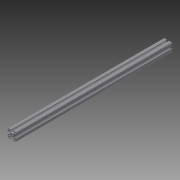
# Autodesk Inventor part: 28 piece
Saved by Autodesk Inventor 2013 (Build 170138000, 138)
## iProperties
Created: 2012-08-14
Part Number: 28 piece
Material: Generic
Document SubType Name: Modeling
Designer: Admin
Density: 1 g/cm^3
Author: Admin
Autodesk Inventor part; units mm, degrees
ref_plane "YZ Plane" through (0, 0, 0) normal (1, 0, 0) x (0, 1, 0)
ref_plane "XZ Plane" through (0, 0, 0) normal (0, 1, 0) x (-1, 0, 0)
ref_plane "XY Plane" through (0, 0, 0) normal (0, 0, 1) x (1, 0, 0)
sketch "Sketch1" plane through (0, 0, 0) normal (0, 0, 1) x (1, 0, 0)
  line L0 (19.5541, -5.1054) -> (14.9059, -5.1054)
  arc A0 (19.9351, -5.4864) -> (19.5541, -5.1054) centre (19.5541, -5.4864) ccw
  line L1 (19.9351, -7.7216) -> (19.9351, -5.4864)
  arc A1 (17.1411, -10.5156) -> (19.9351, -7.7216) centre (17.1411, -7.7216) ccw
  line L2 (14.9059, -10.5156) -> (17.1411, -10.5156)
  arc A2 (14.5249, -10.1346) -> (14.9059, -10.5156) centre (14.9059, -10.1346) ccw
  line L3 (14.5249, -5.4864) -> (14.5249, -10.1346)
  arc A3 (14.9059, -5.1054) -> (14.5249, -5.4864) centre (14.9059, -5.4864) ccw
  arc A4 (5.9905, 6.7564) -> (-0.6643, 6.7564) centre (2.6631, 6.7564) ccw
  arc A5 (-0.6643, 6.7564) -> (5.9905, 6.7564) centre (2.6631, 6.7564) ccw
  line L4 (17.1411, 24.0284) -> (14.9059, 24.0284)
  arc A6 (19.9351, 21.2344) -> (17.1411, 24.0284) centre (17.1411, 21.2344) ccw
  line L5 (19.9351, 18.9992) -> (19.9351, 21.2344)
  arc A7 (19.5541, 18.6182) -> (19.9351, 18.9992) centre (19.5541, 18.9992) ccw
  line L6 (14.9059, 18.6182) -> (19.5541, 18.6182)
  arc A8 (14.5249, 18.9992) -> (14.9059, 18.6182) centre (14.9059, 18.9992) ccw
  line L7 (14.5249, 23.6474) -> (14.5249, 18.9992)
  arc A9 (14.9059, 24.0284) -> (14.5249, 23.6474) centre (14.9059, 23.6474) ccw
  line L8 (-11.8149, -10.5156) -> (-9.5797, -10.5156)
  arc A10 (-14.6089, -7.7216) -> (-11.8149, -10.5156) centre (-11.8149, -7.7216) ccw
  line L9 (-14.6089, -5.4864) -> (-14.6089, -7.7216)
  arc A11 (-14.2279, -5.1054) -> (-14.6089, -5.4864) centre (-14.2279, -5.4864) ccw
  line L10 (-9.5797, -5.1054) -> (-14.2279, -5.1054)
  arc A12 (-9.1987, -5.4864) -> (-9.5797, -5.1054) centre (-9.5797, -5.4864) ccw
  line L11 (-9.1987, -10.1346) -> (-9.1987, -5.4864)
  arc A13 (-9.5797, -10.5156) -> (-9.1987, -10.1346) centre (-9.5797, -10.1346) ccw
  line L12 (-14.2279, 18.6182) -> (-9.5797, 18.6182)
  arc A14 (-14.6089, 18.9992) -> (-14.2279, 18.6182) centre (-14.2279, 18.9992) ccw
  line L13 (-14.6089, 21.2344) -> (-14.6089, 18.9992)
  arc A15 (-11.8149, 24.0284) -> (-14.6089, 21.2344) centre (-11.8149, 21.2344) ccw
  line L14 (-9.5797, 24.0284) -> (-11.8149, 24.0284)
  arc A16 (-9.1987, 23.6474) -> (-9.5797, 24.0284) centre (-9.5797, 23.6474) ccw
  line L15 (-9.1987, 18.9992) -> (-9.1987, 23.6474)
  arc A17 (-9.5797, 18.6182) -> (-9.1987, 18.9992) centre (-9.5797, 18.9992) ccw
  arc A18 (-7.6239, 19.5366) -> (-7.3636, 18.9083) centre (-6.7353, 19.5366) ccw
  line L16 (-7.6239, 19.5366) -> (-7.6239, 21.3111)
  arc A19 (-6.3539, 22.5811) -> (-7.6239, 21.3111) centre (-6.3539, 21.3111) ccw
  line L17 (-6.3539, 22.5811) -> (-4.151, 22.5811)
  line L18 (-4.151, 22.5811) -> (-4.151, 21.7424)
  line L19 (-4.151, 21.7424) -> (-2.9757, 21.7424)
  arc A20 (-2.9757, 21.7424) -> (-1.4009, 23.3172) centre (-2.9757, 23.3172) ccw
  line L20 (-1.4009, 23.3172) -> (-1.4009, 24.2316)
  arc A21 (-1.4009, 24.2316) -> (-2.9757, 25.8064) centre (-2.9757, 24.2316) ccw
  line L21 (-2.9757, 25.8064) -> (-5.3125, 25.8064)
  arc A22 (-6.8365, 25.8064) -> (-5.3125, 25.8064) centre (-6.0745, 25.8064) ccw
  line L22 (-6.8365, 25.8064) -> (-11.6625, 25.8064)
  arc A23 (-13.1865, 25.8064) -> (-11.6625, 25.8064) centre (-12.4245, 25.8064) ccw
  line L23 (-13.1865, 25.8064) -> (-13.2119, 25.8064)
  arc A24 (-13.2119, 25.8064) -> (-16.3869, 22.6314) centre (-13.2119, 22.6314) ccw
  line L24 (-16.3869, 22.6314) -> (-16.3869, 22.606)
  arc A25 (-15.6249, 21.844) -> (-16.3869, 22.606) centre (-16.3869, 21.844) ccw
  arc A26 (-16.3869, 21.082) -> (-15.6249, 21.844) centre (-16.3869, 21.844) ccw
  line L25 (-16.3869, 21.082) -> (-16.3869, 16.256)
  arc A27 (-15.6249, 15.494) -> (-16.3869, 16.256) centre (-16.3869, 15.494) ccw
  arc A28 (-16.3869, 14.732) -> (-15.6249, 15.494) centre (-16.3869, 15.494) ccw
  line L26 (-16.3869, 14.732) -> (-16.3869, 12.3952)
  arc A29 (-16.3869, 12.3952) -> (-14.8121, 10.8204) centre (-14.8121, 12.3952) ccw
  line L27 (-14.8121, 10.8204) -> (-13.8977, 10.8204)
  arc A30 (-13.8977, 10.8204) -> (-12.3229, 12.3952) centre (-13.8977, 12.3952) ccw
  line L28 (-12.3229, 12.3952) -> (-12.3229, 13.507)
  line L29 (-12.3229, 13.507) -> (-13.2159, 13.507)
  line L30 (-13.2159, 13.507) -> (-13.2159, 15.6756)
  arc A31 (-11.9459, 16.9456) -> (-13.2159, 15.6756) centre (-11.9459, 15.6756) ccw
  line L31 (-11.9459, 16.9456) -> (-10.0797, 16.9456)
  arc A32 (-9.4511, 16.6853) -> (-10.0797, 16.9456) centre (-10.0797, 16.0566) ccw
  line L32 (-9.4511, 16.6853) -> (-5.4847, 12.7196)
  arc A33 (-4.0933, 9.3607) -> (-5.4847, 12.7196) centre (-8.8431, 9.3607) ccw
  line L33 (-4.0933, 9.3607) -> (-4.0933, 4.1521)
  arc A34 (-5.4847, 0.7932) -> (-4.0933, 4.1521) centre (-8.8431, 4.1521) ccw
  line L34 (-5.4847, 0.7932) -> (-9.4511, -3.1725)
  arc A35 (-10.0797, -3.4328) -> (-9.4511, -3.1725) centre (-10.0797, -2.5438) ccw
  line L35 (-10.0797, -3.4328) -> (-11.9459, -3.4328)
  arc A36 (-13.2159, -2.1628) -> (-11.9459, -3.4328) centre (-11.9459, -2.1628) ccw
  line L36 (-13.2159, -2.1628) -> (-13.2159, 0.0058)
  line L37 (-13.2159, 0.0058) -> (-12.3229, 0.0058)
  line L38 (-12.3229, 0.0058) -> (-12.3229, 1.1176)
  arc A37 (-12.3229, 1.1176) -> (-13.8977, 2.6924) centre (-13.8977, 1.1176) ccw
  line L39 (-13.8977, 2.6924) -> (-14.8121, 2.6924)
  arc A38 (-14.8121, 2.6924) -> (-16.3869, 1.1176) centre (-14.8121, 1.1176) ccw
  line L40 (-16.3869, 1.1176) -> (-16.3869, -1.2192)
  arc A39 (-15.6249, -1.9812) -> (-16.3869, -1.2192) centre (-16.3869, -1.9812) ccw
  arc A40 (-16.3869, -2.7432) -> (-15.6249, -1.9812) centre (-16.3869, -1.9812) ccw
  line L41 (-16.3869, -2.7432) -> (-16.3869, -7.5692)
  arc A41 (-15.6249, -8.3312) -> (-16.3869, -7.5692) centre (-16.3869, -8.3312) ccw
  arc A42 (-16.3869, -9.0932) -> (-15.6249, -8.3312) centre (-16.3869, -8.3312) ccw
  line L42 (-16.3869, -9.0932) -> (-16.3869, -9.1186)
  arc A43 (-16.3869, -9.1186) -> (-13.2119, -12.2936) centre (-13.2119, -9.1186) ccw
  line L43 (-13.2119, -12.2936) -> (-13.1865, -12.2936)
  arc A44 (-11.6625, -12.2936) -> (-13.1865, -12.2936) centre (-12.4245, -12.2936) ccw
  line L44 (-11.6625, -12.2936) -> (-6.8365, -12.2936)
  arc A45 (-5.3125, -12.2936) -> (-6.8365, -12.2936) centre (-6.0745, -12.2936) ccw
  line L45 (-5.3125, -12.2936) -> (-2.9757, -12.2936)
  arc A46 (-2.9757, -12.2936) -> (-1.4009, -10.7188) centre (-2.9757, -10.7188) ccw
  line L46 (-1.4009, -10.7188) -> (-1.4009, -9.8044)
  arc A47 (-1.4009, -9.8044) -> (-2.9757, -8.2296) centre (-2.9757, -9.8044) ccw
  line L47 (-2.9757, -8.2296) -> (-4.151, -8.2296)
  line L48 (-4.151, -8.2296) -> (-4.151, -9.0683)
  line L49 (-4.151, -9.0683) -> (-6.3539, -9.0683)
  arc A48 (-7.6239, -7.7983) -> (-6.3539, -9.0683) centre (-6.3539, -7.7983) ccw
  line L50 (-7.6239, -7.7983) -> (-7.6239, -6.0238)
  arc A49 (-7.3636, -5.3955) -> (-7.6239, -6.0238) centre (-6.7353, -6.0238) ccw
  line L51 (-7.3636, -5.3955) -> (-3.3583, -1.3909)
  arc A50 (0, 0) -> (-3.3583, -1.3909) centre (0, -4.7498) ccw
  line L52 (0, 0) -> (5.3262, 0)
  arc A51 (8.6846, -1.3909) -> (5.3262, 0) centre (5.3262, -4.7498) ccw
  line L53 (8.6846, -1.3909) -> (12.6898, -5.3955)
  arc A52 (12.9501, -6.0238) -> (12.6898, -5.3955) centre (12.0616, -6.0238) ccw
  line L54 (12.9501, -6.0238) -> (12.9501, -7.7983)
  arc A53 (11.6801, -9.0683) -> (12.9501, -7.7983) centre (11.6801, -7.7983) ccw
  line L55 (11.6801, -9.0683) -> (9.4773, -9.0683)
  line L56 (9.4773, -9.0683) -> (9.4773, -8.2296)
  line L57 (9.4773, -8.2296) -> (8.3019, -8.2296)
  arc A54 (8.3019, -8.2296) -> (6.7271, -9.8044) centre (8.3019, -9.8044) ccw
  line L58 (6.7271, -9.8044) -> (6.7271, -10.7188)
  arc A55 (6.7271, -10.7188) -> (8.3019, -12.2936) centre (8.3019, -10.7188) ccw
  line L59 (8.3019, -12.2936) -> (10.6387, -12.2936)
  arc A56 (12.1627, -12.2936) -> (10.6387, -12.2936) centre (11.4007, -12.2936) ccw
  line L60 (12.1627, -12.2936) -> (16.9887, -12.2936)
  arc A57 (18.5127, -12.2936) -> (16.9887, -12.2936) centre (17.7507, -12.2936) ccw
  line L61 (18.5127, -12.2936) -> (18.5381, -12.2936)
  arc A58 (18.5381, -12.2936) -> (21.7131, -9.1186) centre (18.5381, -9.1186) ccw
  line L62 (21.7131, -9.1186) -> (21.7131, -9.0932)
  arc A59 (21.7131, -7.5692) -> (21.7131, -9.0932) centre (21.7131, -8.3312) ccw
  line L63 (21.7131, -7.5692) -> (21.7131, -2.7432)
  arc A60 (21.7131, -1.2192) -> (21.7131, -2.7432) centre (21.7131, -1.9812) ccw
  line L64 (21.7131, -1.2192) -> (21.7131, 1.1176)
  arc A61 (21.7131, 1.1176) -> (20.1383, 2.6924) centre (20.1383, 1.1176) ccw
  line L65 (20.1383, 2.6924) -> (19.2239, 2.6924)
  arc A62 (19.2239, 2.6924) -> (17.6491, 1.1176) centre (19.2239, 1.1176) ccw
  line L66 (17.6491, 1.1176) -> (17.6491, 0.0058)
  line L67 (17.6491, 0.0058) -> (18.5422, 0.0058)
  line L68 (18.5422, 0.0058) -> (18.5422, -2.1628)
  arc A63 (17.2722, -3.4328) -> (18.5422, -2.1628) centre (17.2722, -2.1628) ccw
  line L69 (17.2722, -3.4328) -> (15.4059, -3.4328)
  arc A64 (14.7773, -3.1725) -> (15.4059, -3.4328) centre (15.4059, -2.5438) ccw
  line L70 (14.7773, -3.1725) -> (10.811, 0.7932)
  arc A65 (9.4195, 4.1521) -> (10.811, 0.7932) centre (14.1693, 4.1521) ccw
  line L71 (9.4195, 4.1521) -> (9.4195, 9.3607)
  arc A66 (10.811, 12.7196) -> (9.4195, 9.3607) centre (14.1693, 9.3607) ccw
  line L72 (10.811, 12.7196) -> (14.7773, 16.6853)
  arc A67 (15.4059, 16.9456) -> (14.7773, 16.6853) centre (15.4059, 16.0566) ccw
  line L73 (15.4059, 16.9456) -> (17.2722, 16.9456)
  arc A68 (18.5422, 15.6756) -> (17.2722, 16.9456) centre (17.2722, 15.6756) ccw
  line L74 (18.5422, 15.6756) -> (18.5422, 13.507)
  line L75 (18.5422, 13.507) -> (17.6491, 13.507)
  line L76 (17.6491, 13.507) -> (17.6491, 12.3952)
  arc A69 (17.6491, 12.3952) -> (19.2239, 10.8204) centre (19.2239, 12.3952) ccw
  line L77 (19.2239, 10.8204) -> (20.1383, 10.8204)
  arc A70 (20.1383, 10.8204) -> (21.7131, 12.3952) centre (20.1383, 12.3952) ccw
  line L78 (21.7131, 12.3952) -> (21.7131, 14.732)
  arc A71 (21.7131, 16.256) -> (21.7131, 14.732) centre (21.7131, 15.494) ccw
  line L79 (21.7131, 16.256) -> (21.7131, 21.082)
  arc A72 (21.7131, 22.606) -> (21.7131, 21.082) centre (21.7131, 21.844) ccw
  line L80 (21.7131, 22.606) -> (21.7131, 22.6314)
  arc A73 (21.7131, 22.6314) -> (18.5381, 25.8064) centre (18.5381, 22.6314) ccw
  line L81 (18.5381, 25.8064) -> (18.5127, 25.8064)
  arc A74 (16.9887, 25.8064) -> (18.5127, 25.8064) centre (17.7507, 25.8064) ccw
  line L82 (16.9887, 25.8064) -> (12.1627, 25.8064)
  arc A75 (10.6387, 25.8064) -> (12.1627, 25.8064) centre (11.4007, 25.8064) ccw
  line L83 (10.6387, 25.8064) -> (8.3019, 25.8064)
  arc A76 (8.3019, 25.8064) -> (6.7271, 24.2316) centre (8.3019, 24.2316) ccw
  line L84 (6.7271, 24.2316) -> (6.7271, 23.3172)
  arc A77 (6.7271, 23.3172) -> (8.3019, 21.7424) centre (8.3019, 23.3172) ccw
  line L85 (8.3019, 21.7424) -> (9.4773, 21.7424)
  line L86 (9.4773, 21.7424) -> (9.4773, 22.5811)
  line L87 (9.4773, 22.5811) -> (11.6801, 22.5811)
  arc A78 (12.9501, 21.3111) -> (11.6801, 22.5811) centre (11.6801, 21.3111) ccw
  line L88 (12.9501, 21.3111) -> (12.9501, 19.5366)
  arc A79 (12.6898, 18.9083) -> (12.9501, 19.5366) centre (12.0616, 19.5366) ccw
  line L89 (12.6898, 18.9083) -> (8.6846, 14.9037)
  arc A80 (5.3262, 13.5128) -> (8.6846, 14.9037) centre (5.3262, 18.2626) ccw
  line L90 (5.3262, 13.5128) -> (0, 13.5128)
  arc A81 (-3.3583, 14.9037) -> (0, 13.5128) centre (0, 18.2626) ccw
  line L91 (-3.3583, 14.9037) -> (-7.3636, 18.9083)
  constraints: 184 end point, 164 point on circle, 82 centre point
extrude "Extrusion1" add sketch "Sketch1" along normal blind 711.2
body "Solid1"
